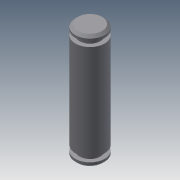
# Autodesk Inventor part: hridelka1
Saved by Autodesk Inventor 2013 (Build 170138000, 138)
## iProperties
Created: 2013-05-13
Part Number: hridelka1
Material: Generic
Document SubType Name: Modeling
Designer: idle-rug
Density: 1 g/cm^3
Author: idle-rug
Autodesk Inventor part; units mm, degrees
ref_plane "YZ Plane" through (0, 0, 0) normal (1, 0, 0) x (0, 1, 0)
ref_plane "XZ Plane" through (0, 0, 0) normal (0, 1, 0) x (-1, 0, 0)
ref_plane "XY Plane" through (0, 0, 0) normal (0, 0, 1) x (1, 0, 0)
sketch "Sketch1" plane through (0, 0, 0) normal (1, 0, 0) x (0, 1, 0)
  line L0 (0, -12) -> (3, -12)
  line L1 (3, 12) -> (0, 12)
  line L2 (0, 12) -> (0, -12)
  line L3 (3, 9) -> (3, -9)
  line L4 (3, 0) -> (0, 0)
  line L5 (0, -9.75) -> (0, 9.75)
  line L6 (3, 9.75) -> (3, -9.75)
  line L7 (3, 10.75) -> (2.15, 10.75)
  line L8 (2.15, 10.75) -> (2.15, 9.75)
  line L9 (3, 12) -> (3, 10.75)
  line L10 (2.15, 9.75) -> (3, 9.75)
  line L11 (3, -10.75) -> (2.15, -10.75)
  line L12 (2.15, -10.75) -> (2.15, -9.75)
  line L13 (2.15, -9.75) -> (3, -9.75)
  line L14 (3, -10.75) -> (3, -12)
  line L15 (0, -16.8) -> (0, 16.8) projected
  point P0 (1.5, 0)
  dimension "d12" = 19.5
  dimension "d13" = 1
  dimension "d14" = 0.85
  dimension "d16" = 1
  constraints: 30 end point, 3 parallel, 2 midpoint, 2 perpendicular, 1 horizontal, 1 point on line
  measures "d12" distance of L5.start L5.end
  measures "d13" distance of L6.start L7.start
  measures "d14" distance of L7.start L7.end
  measures "d16" distance of L11.end L12.end
revolve "Revolution1" add sketch "Sketch1" angle 360 about axis through (0, 0, -10) along (0, 0, 1)
sketch "Sketch2" plane through (0, 0, 12) normal (0, 0, 1) x (1, 0, 0)
  circle A0 centre (0, 0) radius 3 projected
extrude "Extrusion1" cut sketch "Sketch2" against normal blind 0.25
sketch "Sketch3" plane through (0, 0, -12) normal (0, 0, -1) x (-1, 0, 0)
  circle A0 centre (0, 0) radius 3 projected
extrude "Extrusion2" cut sketch "Sketch3" against normal blind 0.25
chamfer "Chamfer1" distance 0.5 angle 45 2 edges at (0, -3, -11.75) (0, -3, 11.75)
body "Solid1"
